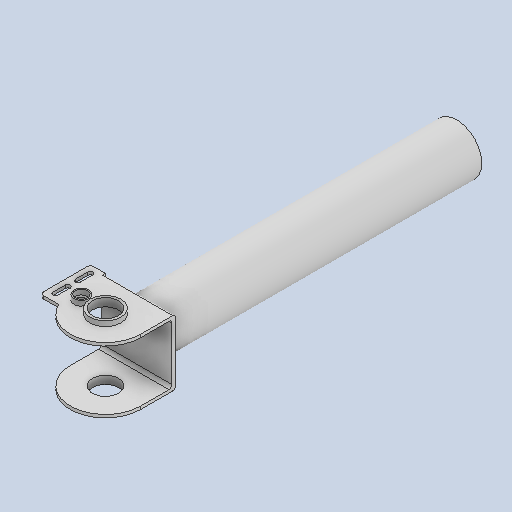
# Autodesk Inventor part: czlon_1
Saved by Autodesk Inventor 2023 (Build 270158000, 158)
## iProperties
Created: 2023-04-01
Part Number: czlon_1
Material: Ogólny
Document SubType Name: Modeling
Designer: krzys
Density: 1 g/cm^3
Appearance: Domyślna
Author: krzys
Autodesk Inventor part; units mm, degrees
ref_plane "YZ Plane" through (0, 0, 0) normal (1, 0, 0) x (0, 1, 0)
ref_plane "XZ Plane" through (0, 0, 0) normal (0, 1, 0) x (-1, 0, 0)
ref_plane "XY Plane" through (0, 0, 0) normal (0, 0, 1) x (1, 0, 0)
sketch "Szkic1" plane through (0, 0, 0) normal (0, 0, 1) x (1, 0, 0)
  circle A0 centre (0, 0) radius 50
  circle A1 centre (0, 0) radius 46
  circle A2 centre (0, 0) radius 31.5
  circle A3 centre (-28.9914, 28.9914) radius 4
  circle A4 centre (-28.9914, -28.9914) radius 4
  circle A5 centre (28.9914, 28.9914) radius 4
  circle A6 centre (28.9914, -28.9914) radius 4
  dimension "d0" = 100
  dimension "d1" = 92
  dimension "d2" = 63
  dimension "d4" = 8
  dimension "d5" = 8
  dimension "d6" = 8
  dimension "d7" = 8
  constraints: 7 centre point, 3 coincident
  measures "d0" diameter of A0
  measures "d1" diameter of A1
  measures "d2" diameter of A2
  measures "d4" diameter of A3
  measures "d5" diameter of A4
  measures "d6" diameter of A5
  measures "d7" diameter of A6
extrude "Wyciągnięcie proste1" add sketch "Szkic1" along normal blind 4 contours A1
extrude "Wyciągnięcie proste2" add sketch "Szkic1" along normal blind 700 contours A0
sketch "Szkic5" plane through (0, 0, 0) normal (0, 1, 0) x (-1, 0, 0)
  line L0 (50, 700) -> (-50, 700) projected
  arc A0 (70, 700) -> (-70, 700) centre (0, 700) ccw
  circle A1 centre (0, 700) radius 26
  circle A2 centre (0, 700) radius 31
  line L1 (0, 630) -> (70, 630)
  line L2 (70, 630) -> (70, 700)
  line L3 (0, 630) -> (-70, 630)
  line L4 (-70, 630) -> (-70, 700)
  line L5 (0, 637.5) -> (70, 637.5)
  line L6 (0, 637.5) -> (-70, 637.5)
  point P0 (0, 0)
  point P1 (26, 700)
  point P2 (-26, 700)
  dimension "d28" = 140
  dimension "d29" = 52
  dimension "d35" = 62
  constraints: 12 end point, 4 point on line, 3 centre point, 2 perpendicular, 2 point on circle, 2 tangent, 1 coincident, 1 horizontal, 1 midpoint
  measures "d28" diameter of A0
  measures "d29" diameter of A1
  measures "d35" diameter of A2
extrude "Wyciągnięcie proste7" add sketch "Szkic5" along normal mid plane 130 contours A2 L0 A1 | L0 A1 A2 | A1 L0 | L0 A1 | L2 L5 L6 L4 A0 | L2 L1 L3 L4 L6 L5
extrude "Wyciągnięcie proste8" cut sketch "Szkic5" along normal mid plane 130 contours A1 L0 | L0 A1
extrude "Wyciągnięcie proste9" add sketch "Szkic5" along normal mid plane 150 contours A2 L0 A1 | L0 A1 A2
extrude "Wyciągnięcie proste10" cut sketch "Szkic5" along normal mid plane 118 contours A2 L0 A1 | L0 A1 A2 | A1 L0 | L0 A1 | L2 L5 L6 L4 A0 | L2 L1 L3 L4 L6 L5
sketch "Szkic7" plane through (0, 65, 700) normal (0, 1, 0) x (1, 0, 0)
  circle A0 centre (-48, 0) radius 7.5
  circle A1 centre (-48, 0) radius 12.5
  circle A2 centre (-48, 0) radius 15
  line L0 (-70, 70) -> (-70, 0) projected
  line L1 (-70, 70) -> (-94, 70)
  line L2 (-100, 64) -> (-100, -24)
  arc A3 (-70, 0) -> (70, 0) centre (0, 0) ccw projected
  line L3 (-94, -30) -> (-63.2456, -30)
  arc A4 (-100, -24) -> (-94, -30) centre (-94, -24) ccw
  arc A5 (-94, 70) -> (-100, 64) centre (-94, 64) ccw
  arc A6 (-80, 55) -> (-90, 55) centre (-85, 55) ccw
  arc A7 (-90, -15) -> (-80, -15) centre (-85, -15) ccw
  arc A8 (-90, 30) -> (-80, 30) centre (-85, 30) ccw
  arc A9 (-80, 10) -> (-90, 10) centre (-85, 10) ccw
  line L4 (-80, 10) -> (-80, -15)
  line L5 (-90, -15) -> (-90, 10)
  line L6 (-80, 55) -> (-80, 30)
  line L7 (-90, 30) -> (-90, 55)
  point P0 (0, 700)
  point P1 (-100, 70)
  point P2 (-100, -30)
  dimension "d46" = 15
  dimension "d47" = 25
  dimension "d48" = 30
  dimension "d57" = 30
  dimension "d58" = 100
  dimension "d59" = 6
  dimension "d60" = 6
  dimension "d62" = 10
  dimension "d63" = 10
  dimension "d64" = 10
  dimension "d66" = 10
  dimension "d67" = 25
  constraints: 14 end point, 13 point on circle, 9 centre point, 8 point on line, 6 tangent, 2 coincident, 2 horizontal, 1 perpendicular
  measures "d46" diameter of A0
  measures "d47" diameter of A1
  measures "d48" diameter of A2
  measures "d57" distance of L0.start point (-100, 70)
  measures "d58" distance of point (-100, 70) point (-100, -30)
  measures "d59" radius of A4
  measures "d60" radius of A5
  measures "d62" diameter of A6
  measures "d63" diameter of A7
  measures "d64" diameter of A8
  measures "d66" diameter of A9
  measures "d67" distance of A7.centre A9.centre
extrude "Wyciągnięcie proste13" add sketch "Szkic7" along normal blind 10 contours A2
extrude "Wyciągnięcie proste14" cut sketch "Szkic7" against normal blind 6 contours A0
extrude "Wyciągnięcie proste15" add sketch "Szkic5" along normal mid plane 130 contours L2 L1 L3 L4 L6 L5
fillet "Zaokrąglenie1" radius 6 4 edges at (0, 65, 630) (0, -65, 630) (0, 59, 637.5) (0, -59, 637.5)
fillet "Zaokrąglenie2" radius 6 1 edges at (-50, 0, 630)
extrude "Wyciągnięcie proste16" add sketch "Szkic7" against normal blind 6 contours L0 A3 L3 A4 L2 A5 L1
